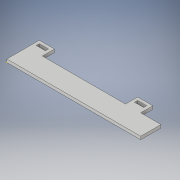
# Autodesk Inventor part: ball-reload-right
Saved by Autodesk Inventor 2017 (Build 210142000, 142)
## iProperties
Created: 2017-03-05
Part Number: ball-reload-right
Material: Generic
Document SubType Name: Modeling
Designer: John
Density: 1 g/cm^3
Appearance: Default
Author: John
Autodesk Inventor part; units mm, degrees
ref_plane "YZ Plane" through (0, 0, 0) normal (1, 0, 0) x (0, 1, 0)
ref_plane "XZ Plane" through (0, 0, 0) normal (0, 1, 0) x (-1, 0, 0)
ref_plane "XY Plane" through (0, 0, 0) normal (0, 0, 1) x (1, 0, 0)
sketch "Sketch1" plane through (0, 0, 0) normal (0, 1, 0) x (-1, 0, 0)
  point P0 (0, 0)
sketch "Sketch2" plane through (0, 0, 0) normal (0, 1, 0) x (-1, 0, 0)
  line L0 (0, 0) -> (-132, 0)
  line L1 (-132, 0) -> (-132, -20)
  line L2 (-132, -20) -> (0, -20)
  line L3 (0, -20) -> (0, 0)
  dimension "d0" = 132
  dimension "d1" = 20
  constraints: 8 end point, 2 parallel, 1 horizontal, 1 perpendicular
  measures "d0" distance of L2.end L1.end
  measures "d1" distance of L1.end L0.end
extrude "Extrusion1" add sketch "Sketch2" along normal blind 3
sketch "Sketch3" plane through (0, 3, 0) normal (0, 1, 0) x (1, 0, 0)
  line L0 (132, 20) -> (0, 20) projected
  line L1 (0, 20) -> (15, 20)
  line L2 (15, 20) -> (15, 32)
  line L3 (15, 32) -> (0, 32)
  line L4 (0, 32) -> (0, 20)
  line L5 (3, 29) -> (12, 29)
  line L6 (12, 29) -> (12, 26)
  line L7 (12, 26) -> (3, 26)
  line L8 (3, 26) -> (3, 29)
  line L9 (132, 0) -> (132, 20)
  line L10 (112, 20) -> (97, 20)
  line L11 (97, 20) -> (97, 32)
  line L12 (97, 32) -> (112, 32)
  line L13 (112, 32) -> (112, 20)
  line L14 (109, 29) -> (100, 29)
  line L15 (100, 29) -> (100, 26)
  line L16 (100, 26) -> (109, 26)
  line L17 (109, 26) -> (109, 29)
  point P0 (0, 0)
  dimension "d4" = 15
  dimension "d8" = 3
  dimension "d9" = 3
  dimension "d10" = 3
  dimension "d11" = 6
  dimension "d12" = 3
  dimension "d13" = 15
  dimension "d14" = 3
  dimension "d15" = 3
  dimension "d16" = 3
  dimension "d17" = 3
  dimension "d18" = 6
  dimension "d19" = 82
  constraints: 34 end point, 8 parallel, 4 horizontal, 4 perpendicular
  measures "d4" distance of L3.end L2.end
  measures "d8" distance between parallel lines of L3 L5
  measures "d9" distance between parallel lines of L2 L6
  measures "d10" distance between parallel lines of L4 L8
  measures "d11" distance between parallel lines of L0 L7
  measures "d12" distance of L5.end L6.end
  measures "d13" distance of L11.end L12.end
  measures "d14" distance of L16.end L14.start
  measures "d15" distance between parallel lines of L12 L14
  measures "d16" distance between parallel lines of L13 L17
  measures "d17" distance between parallel lines of L11 L15
  measures "d18" distance between parallel lines of L0 L16
  measures "d19" distance between parallel lines of L11 L2
extrude "Extrusion2" add sketch "Sketch3" against normal blind 3
equation "\"d9\" = d8"
equation "\"d10\" = d8"
equation "\"d16\" = d15"
equation "\"d17\" = d15"
body "Solid1"
